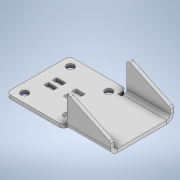
# Autodesk Inventor part: base_cuerpo_chapa
Saved by Autodesk Inventor 2021 (Build 250183000, 183)
## iProperties
Created: 2026-06-23
Part Number: base_cuerpo_chapa
Material: Generic
Document SubType Name: Sheet Metal
Designer: nelso
Density: 1 g/cm^3
Flat Pattern Width: 10.3751 cm
Flat Pattern Length: 9.42 cm
Flat Pattern Area: 97.7335 cm^2
Sheet Metal Rule: Default_mm
Sheet Metal Width: 103.751 mm
Sheet Metal Length: 94.200 mm
Sheet Metal Area: 9773.350 mm^2
Appearance: Default
Author: nelso
Autodesk Inventor part; units mm, degrees
ref_plane "YZ Plane" through (0, 0, 0) normal (1, 0, 0) x (0, 1, 0)
ref_plane "XZ Plane" through (0, 0, 0) normal (0, 1, 0) x (-1, 0, 0)
ref_plane "XY Plane" through (0, 0, 0) normal (0, 0, 1) x (1, 0, 0)
sketch "Sketch1" plane through (0, 0, 0) normal (0, 1, 0) x (-1, 0, 0)
  line L0 (-27.1, 28.6) -> (27.1, 28.6)
  line L1 (27.1, 28.6) -> (27.1, -28.6)
  line L2 (27.1, -28.6) -> (-27.1, -28.6)
  line L3 (-27.1, -28.6) -> (-27.1, 28.6)
  line L4 (-27.1, 28.6) -> (27.1, -28.6) construction
  line L5 (27.1, 28.6) -> (-27.1, -28.6) construction
  line L6 (27.1, 28.6) -> (27.1, 20.7)
  line L7 (27.1, 20.7) -> (18.4, 20.7)
  line L8 (-27.1, 28.6) -> (-18.4, 28.6)
  line L9 (-27.1, 20.7) -> (-27.1, 28.6)
  line L10 (27.1, -28.6) -> (18.4, -28.6)
  line L11 (27.1, -20.7) -> (27.1, -28.6)
  line L12 (-27.1, -28.6) -> (-18.4, -28.6)
  line L13 (-27.1, -20.7) -> (-27.1, -28.6)
  circle A0 centre (18.4, 20.7) radius 3.35
  circle A1 centre (-18.4, 18.6) radius 3.35
  circle A2 centre (-18.4, -18.6) radius 3.35
  circle A3 centre (18.4, -20.7) radius 3.35
  line L14 (-27.1, 28.6) -> (-67.1, 28.6)
  line L15 (-67.1, 28.6) -> (-67.1, -28.6)
  line L16 (-67.1, -28.6) -> (-27.1, -28.6)
  line L17 (-27.1, -28.6) -> (-27.1, 28.6)
  line L18 (-67.1, -28.6) -> (-27.1, -28.6)
  line L19 (-67.1, 28.6) -> (-27.1, 28.6)
  line L20 (27.1, 0) -> (15.9, 0)
  line L21 (15.9, 6.0647) -> (15.9, 0)
  line L22 (15.9, 0) -> (8.4, 0)
  line L23 (8.4, 0) -> (8.4, 6.0647)
  line L24 (8.4, 0) -> (-1.6, 0)
  line L25 (-1.6, 0) -> (-1.6, 5.7069)
  line L26 (-1.6, 0) -> (-9.1, 0)
  line L27 (-9.1, 0) -> (-9.1, 5.7069)
  line L28 (-9.1, 0) -> (-25.3, 0)
  line L29 (-25.3, 0) -> (-25.3, 8.0124)
  line L30 (0, 0) -> (0, 1.4)
  line L31 (0, 0) -> (0, -1.279)
  dimension "d0" = 54.2
  dimension "d1" = 57.2
  dimension "d2" = 7.9
  dimension "d3" = 8.7
  dimension "d10" = 6.7
  dimension "d11" = 6.7
  dimension "d12" = 6.7
  dimension "d13" = 6.7
  dimension "d15" = 57.2
  dimension "d73" = 11.2
  dimension "d74" = 7.5
  dimension "d75" = 10
  dimension "d76" = 7.5
  dimension "d77" = 16.2
  dimension "d78" = 1.4
  dimension "d99" = 10
  dimension "d100" = 10
  measures "d0" distance of L1.end L2.end
  measures "d1" distance of L0.end L1.end
  measures "d2" distance of L0.end L6.end
  measures "d3" distance of L6.end L7.end
  measures "d10" diameter of A0
  measures "d11" diameter of A1
  measures "d12" diameter of A2
  measures "d13" diameter of A3
  measures "d15" distance of L15.end L14.end
  measures "d73" distance of L20.start L20.end
  measures "d74" distance of L20.end L22.end
  measures "d75" distance of L22.end L24.end
  measures "d76" distance of L24.end L26.end
  measures "d77" distance of L26.end L28.end
  measures "d78" distance of L30.start L30.end
  measures "d99" distance from line of L0 A1.centre
  measures "d100" distance from line of L2 A2.centre
extrude "Plate1" add sketch "Sketch1" along normal blind 3.2
sketch "Sketch5" plane through (67.1, 0, 25.4) normal (0, 0, 1) x (1, 0, 0)
  line L0 (-39.2, 0) -> (0, 0)
  line L1 (0, 0) -> (0, 30)
  line L2 (0, 30) -> (-39.2, 30)
  line L3 (-39.2, 30) -> (-39.2, 0)
  constraints: 6 end point, 1 horizontal, 1 perpendicular, 1 vertical
edge flange "Flange3" height 30 angle 90 thickness 3.2 bend radius 3.2 thickness toward (0, 0, 1) relief straight relief width 3.2 relief depth 1.6 edges at (20, 3.2, 28.6) wall of the first edge with corners at (27.9, 0, 25.4) (67.1, 0, 25.4) (67.1, 30, 25.4) (27.9, 30, 25.4)
bend "Bend3"
corner "Corner3"
sketch "Sketch6" plane through (-27.1, 0, -25.4) normal (0, 0, -1) x (-1, 0, 0)
  line L0 (-94.2, 0) -> (-55, 0)
  line L1 (-55, 0) -> (-55, 30)
  line L2 (-55, 30) -> (-94.2, 30)
  line L3 (-94.2, 30) -> (-94.2, 0)
  constraints: 8 end point
edge flange "Flange4" height 30 angle 90 thickness 3.2 bend radius 3.2 thickness toward (0, 0, -1) relief straight relief width 3.2 relief depth 1.6 edges at (20, 3.2, -28.6) wall of the first edge with corners at (67.1, 0, -25.4) (27.9, 0, -25.4) (27.9, 30, -25.4) (67.1, 30, -25.4)
bend "Bend4"
corner "Corner4"
sketch "Sketch11" plane through (0, 3.2, 0) normal (0, 1, 0) x (1, 0, 0)
  line L0 (-15.9, 1.75) -> (-15.9, 4.95)
  line L1 (-15.9, 4.95) -> (-8.4, 4.95)
  line L2 (-8.4, 4.95) -> (-8.4, 1.75)
  line L3 (-8.4, 1.75) -> (-15.9, 1.75)
  line L4 (1.6, 1.75) -> (1.6, 4.95)
  line L5 (1.6, 4.95) -> (9.1, 4.95)
  line L6 (9.1, 4.95) -> (9.1, 1.75)
  line L7 (9.1, 1.75) -> (1.6, 1.75)
  line L8 (-15.9, -4.95) -> (-15.9, -1.75)
  line L9 (-15.9, -1.75) -> (-8.4, -1.75)
  line L10 (-8.4, -1.75) -> (-8.4, -4.95)
  line L11 (-8.4, -4.95) -> (-15.9, -4.95)
  line L12 (1.6, -4.95) -> (1.6, -1.75)
  line L13 (1.6, -1.75) -> (9.1, -1.75)
  line L14 (9.1, -1.75) -> (9.1, -4.95)
  line L15 (9.1, -4.95) -> (1.6, -4.95)
  line L16 (-15.9, 1.75) -> (-7.6, 1.75)
  line L17 (-7.6, 1.75) -> (-7.6, 5.75)
  line L18 (-7.6, 5.75) -> (-15.9, 5.75)
  line L19 (-15.9, 5.75) -> (-15.9, 1.75)
  line L20 (-15.9, -1.75) -> (-7.6, -1.75)
  line L21 (-7.6, -1.75) -> (-7.6, -5.75)
  line L22 (-7.6, -5.75) -> (-15.9, -5.75)
  line L23 (-15.9, -5.75) -> (-15.9, -1.75)
  line L24 (1.6, -1.75) -> (9.9, -1.75)
  line L25 (9.9, -1.75) -> (9.9, -5.75)
  line L26 (9.9, -5.75) -> (1.6, -5.75)
  line L27 (1.6, -5.75) -> (1.6, -1.75)
  line L28 (1.6, 1.75) -> (9.9, 1.75)
  line L29 (9.9, 1.75) -> (9.9, 5.75)
  line L30 (9.9, 5.75) -> (1.6, 5.75)
  line L31 (1.6, 5.75) -> (1.6, 1.75)
  point P0 (0, 0)
  dimension "d89" = 8.3
  dimension "d90" = 4
  dimension "d91" = 8.3
  dimension "d92" = 4
  dimension "d93" = 8.3
  dimension "d94" = 4
  dimension "d95" = 8.3
  dimension "d96" = 4
  constraints: 64 end point, 12 horizontal, 8 parallel, 8 vertical, 4 perpendicular, 16 other
  measures "d89" distance of L18.end L17.end
  measures "d90" distance of L17.end L16.end
  measures "d91" distance of L21.end L22.end
  measures "d92" distance of L20.end L21.end
  measures "d93" distance of L25.end L26.end
  measures "d94" distance of L24.end L25.end
  measures "d95" distance of L30.end L29.end
  measures "d96" distance of L29.end L28.end
extrude "Cut3" cut sketch "Sketch11" against normal blind 3.2
fillet "Corner Round1" radius 4 4 edges at (-27.1, 1.6, -28.6) (-27.1, 1.6, 28.6) (24.7, 1.6, 28.6) (24.7, 1.6, -28.6)
sketch "Sketch12" plane through (67.1, 30, -28.6) normal (0, 0, -1) x (-1, 0, 0)
  line L0 (0, -23.6) -> (39.2, -23.6) projected
  line L1 (0, -23.6) -> (0, -18.6)
  line L2 (0, 0) -> (0, -23.6) projected
  line L3 (39.2, 0) -> (0, 0) projected
  line L4 (0, -18.6) -> (39.2, 0)
  line L5 (39.2, 0) -> (39.2, -18.6)
  line L6 (39.2, -23.6) -> (39.2, 0) projected
  line L7 (0, -18.6) -> (39.2, -18.6)
  point P0 (67.1, -30)
  dimension "d102" = 5
  constraints: 8 end point, 2 point on line, 1 perpendicular
  measures "d102" distance of L0.start L1.end
extrude "Cut4" cut sketch "Sketch12" against normal up to surface (57.2 mm away) contours L2 L3 L4
fillet "Corner Round2" radius 2 4 edges at (27.9, 30, 27) (27.9, 30, -27) (67.1, 11.4, 27) (67.1, 11.4, -27)
equation "\"d100\" = d99"
equation "\"d89\" = d91"
equation "\"d90\" = d92"
equation "\"d93\" = d91"
equation "\"d94\" = d92"
equation "\"d95\" = d91"
equation "\"d96\" = d92"
equation "\"d97\" = Thickness"
equation "\"d103\" = Thickness"
equation "\"d22\" = Thickness"
equation "\"d49\" = BendReliefWidth"
equation "\"d50\" = BendReliefDepth"
equation "\"d51\" = MinimumRemnant"
equation "\"d52\" = TransitionRadius"
equation "\"d57\" = BendRadius"
equation "\"d58\" = CornerReliefSize"
equation "\"d59\" = GapSize"
equation "\"d60\" = JacobiRadiusSize"
equation "\"d61\" = BendReliefWidth"
equation "\"d62\" = BendReliefDepth"
equation "\"d63\" = MinimumRemnant"
equation "\"d64\" = TransitionRadius"
equation "\"d69\" = BendRadius"
equation "\"d70\" = CornerReliefSize"
equation "\"d71\" = GapSize"
equation "\"d72\" = JacobiRadiusSize"
equation "\"BendRadius\" = Thickness"
equation "\"BendReliefWidth\" = Thickness"
equation "\"BendReliefDepth\" = 0.5 * Thickness"
equation "\"CornerReliefSize\" = 4 * Thickness"
equation "\"MinimumRemnant\" = 2 * Thickness"
equation "\"TransitionRadius\" = BendRadius"
equation "\"JacobiRadiusSize\" = BendRadius"
equation "\"GapSize\" = Thickness"
equation "\"Thickness\" = 3.2"
body "Solid1"
